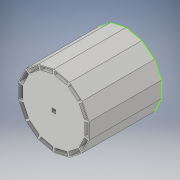
# Autodesk Inventor part: Magnetic Revolver
Saved by Autodesk Inventor 2018.3 (Build 223284000, 284)
## iProperties
Created: 2019-01-14
Part Number: Magnetic Revolver
Material: Generic
Document SubType Name: Modeling
Designer: locuser
Density: 1 g/cm^3
Appearance: Default
Author: locuser
Autodesk Inventor part; units mm, degrees
ref_plane "YZ Plane" through (0, 0, 0) normal (1, 0, 0) x (0, 1, 0)
ref_plane "XZ Plane" through (0, 0, 0) normal (0, 1, 0) x (-1, 0, 0)
ref_plane "XY Plane" through (0, 0, 0) normal (0, 0, 1) x (1, 0, 0)
sketch "Sketch1" plane through (0, 0, 0) normal (0, 0, 1) x (1, 0, 0)
  line L0 (0, 31.75) -> (13.7758, 28.6058)
  line L1 (13.7758, 28.6058) -> (24.8231, 19.7958)
  line L2 (24.8231, 19.7958) -> (30.954, 7.065)
  line L3 (30.954, 7.065) -> (30.954, -7.065)
  line L4 (30.954, -7.065) -> (24.8231, -19.7958)
  line L5 (24.8231, -19.7958) -> (13.7758, -28.6058)
  line L6 (13.7758, -28.6058) -> (0, -31.75)
  line L7 (0, -31.75) -> (-13.7758, -28.6058)
  line L8 (-13.7758, -28.6058) -> (-24.8231, -19.7958)
  line L9 (-24.8231, -19.7958) -> (-30.954, -7.065)
  line L10 (-30.954, -7.065) -> (-30.954, 7.065)
  line L11 (-30.954, 7.065) -> (-24.8231, 19.7958)
  line L12 (-24.8231, 19.7958) -> (-13.7758, 28.6058)
  line L13 (-13.7758, 28.6058) -> (0, 31.75)
  point P0 (0, 0)
  point P1 (0, 0)
  constraints: 28 end point, 1 coincident, 29 other
extrude "Extrusion1" add sketch "Sketch1" along normal blind 63.5
sketch "Sketch3" plane through (0, 0, 0) normal (0, 0, -1) x (-1, 0, 0)
  line L0 (0, -1.5875) -> (1.5875, -1.5875)
  line L1 (1.5875, -1.5875) -> (-1.5875, -1.5875)
  line L2 (1.5875, -1.5875) -> (-1.5875, -1.5875)
  line L3 (-1.5875, -1.5875) -> (-1.5875, 1.5921)
  line L4 (-1.5875, 1.5921) -> (1.5875, 1.5921)
  line L5 (1.5875, 1.5921) -> (1.5875, -1.5875)
  point P0 (0, 0)
  constraints: 12 end point, 2 horizontal, 2 parallel, 1 perpendicular, 1 point on line
extrude "Extrusion3" cut sketch "Sketch3" against normal blind 63.5
sketch "Sketch4" plane through (0, 0, 0) normal (0, 0, -1) x (-1, 0, 0)
  line L0 (-13.7758, 28.6058) -> (0, 31.75) projected
  line L1 (0, 0) -> (0, 31.75)
  line L2 (0, 31.75) -> (0, 0)
  line L3 (0, 26.7538) -> (11.6081, 24.1044)
  line L4 (11.6081, 24.1044) -> (20.917, 16.6807)
  line L5 (20.917, 16.6807) -> (26.0831, 5.9533)
  line L6 (26.0831, 5.9533) -> (26.0831, -5.9533)
  line L7 (26.0831, -5.9533) -> (20.917, -16.6807)
  line L8 (20.917, -16.6807) -> (11.6081, -24.1044)
  line L9 (11.6081, -24.1044) -> (0, -26.7538)
  line L10 (0, -26.7538) -> (-11.6081, -24.1044)
  line L11 (-11.6081, -24.1044) -> (-20.917, -16.6807)
  line L12 (-20.917, -16.6807) -> (-26.0831, -5.9533)
  line L13 (-26.0831, -5.9533) -> (-26.0831, 5.9533)
  line L14 (-26.0831, 5.9533) -> (-20.917, 16.6807)
  line L15 (-20.917, 16.6807) -> (-11.6081, 24.1044)
  line L16 (-11.6081, 24.1044) -> (0, 26.7538)
  line L17 (-10.8414, 24.2794) -> (-13.0091, 28.7808)
  line L18 (-14.3715, 28.0758) -> (-12.2229, 23.6141)
  constraints: 36 end point, 4 point on line, 2 coincident, 1 collinear, 1 parallel, 1 vertical, 29 other
sketch "Sketch5" plane through (0, 0, 63.5) normal (0, 0, 1) x (1, 0, 0)
  line L0 (0.8565, 27.7445) -> (0.8565, 30.7925)
  line L1 (-0.9215, 30.7777) -> (-0.9215, 27.7297)
  line L2 (-12.5635, 26.0885) -> (-13.3645, 25.7027) construction
  line L3 (-11.2337, 25.376) -> (-12.5635, 28.1205)
  line L4 (-14.164, 27.346) -> (-12.8356, 24.6045)
  line L5 (-22.6387, 18.0538) -> (-23.193, 17.3587) construction
  line L6 (-21.1314, 17.9888) -> (-23.5145, 19.8892)
  line L7 (-24.623, 18.4991) -> (-22.24, 16.5987)
  line L8 (-28.23, 6.4433) -> (-28.4278, 5.5766) construction
  line L9 (-30.2111, 5.9601) -> (-27.2395, 5.2819)
  line L10 (-28.23, -6.4433) -> (-28.4278, -5.5766) construction
  line L11 (-26.8318, -7.0637) -> (-29.8154, -7.717)
  line L12 (-30.2111, -5.9836) -> (-27.2395, -5.333)
  line L13 (12.5635, 26.0885) -> (11.7625, 26.474) construction
  line L14 (12.8362, 24.6041) -> (14.1581, 27.3507)
  line L15 (12.5562, 28.1221) -> (11.2344, 25.3758)
  line L16 (22.6387, 18.0538) -> (22.0844, 18.7488) construction
  line L17 (22.24, 16.5987) -> (24.623, 18.4991)
  line L18 (23.5145, 19.8892) -> (21.1314, 17.9888)
  line L19 (28.23, 6.4433) -> (28.0322, 7.31) construction
  line L20 (27.2395, 5.2855) -> (30.2111, 5.9836)
  line L21 (29.8154, 7.717) -> (26.8524, 7.021)
  line L22 (27.2481, -6.2448) -> (27.4459, -5.3781) construction
  line L23 (22.6387, -18.0538) -> (23.193, -17.3587) construction
  line L24 (21.1314, -17.9888) -> (23.5145, -19.8892)
  line L25 (24.623, -18.4991) -> (22.24, -16.5987)
  line L26 (12.5635, -26.0885) -> (13.3645, -25.7027) construction
  line L27 (11.2433, -25.3738) -> (12.533, -28.1274)
  line L28 (14.1215, -27.3799) -> (12.8255, -24.6126)
  line L29 (0, -28.956) -> (-0.889, -28.956) construction
  line L30 (0.8793, -27.7393) -> (0.8793, -30.7873)
  line L31 (-0.8987, -30.7829) -> (-0.8987, -27.7349)
  line L32 (-12.5635, -26.0885) -> (-13.3645, -25.7027) construction
  line L33 (-12.8255, -24.6126) -> (-12.8255, -24.6126)
  line L34 (-11.2433, -25.3738) -> (-12.5601, -28.1212)
  line L35 (-14.148, -27.3602) -> (-14.1434, -27.3624)
  line L36 (-14.1434, -27.3624) -> (-12.8255, -24.6126)
  line L37 (-22.6387, -18.0538) -> (-23.193, -17.3587) construction
  line L38 (-21.1314, -17.9888) -> (-23.5145, -19.8892)
  line L39 (-24.623, -18.4991) -> (-22.24, -16.5987)
  line L40 (0, 30.988) -> (13.4452, 27.9192)
  line L41 (13.4452, 27.9192) -> (24.2274, 19.3207)
  line L42 (24.2274, 19.3207) -> (30.2111, 6.8955)
  line L43 (30.2111, 6.8955) -> (30.2111, -6.8955)
  line L44 (30.2111, -6.8955) -> (24.2274, -19.3207)
  line L45 (24.2274, -19.3207) -> (13.4452, -27.9192)
  line L46 (13.4452, -27.9192) -> (0, -30.988)
  line L47 (0, -30.988) -> (-13.4452, -27.9192)
  line L48 (-13.4452, -27.9192) -> (-24.2274, -19.3207)
  line L49 (-24.2274, -19.3207) -> (-30.2111, -6.8955)
  line L50 (-30.2111, -6.8955) -> (-30.2111, 6.8955)
  line L51 (-30.2111, 6.8955) -> (-24.2274, 19.3207)
  line L52 (-24.2274, 19.3207) -> (-13.4452, 27.9192)
  line L53 (-13.4452, 27.9192) -> (0, 30.988)
  line L54 (0, 27.94) -> (12.1227, 25.1731)
  line L55 (12.1227, 25.1731) -> (21.8444, 17.4203)
  line L56 (21.8444, 17.4203) -> (27.2395, 6.2172)
  line L57 (27.2395, 6.2172) -> (27.2395, -6.2172)
  line L58 (27.2395, -6.2172) -> (21.8444, -17.4203)
  line L59 (21.8444, -17.4203) -> (12.1227, -25.1731)
  line L60 (12.1227, -25.1731) -> (0, -27.94)
  line L61 (0, -27.94) -> (-12.1227, -25.1731)
  line L62 (-12.1227, -25.1731) -> (-21.8444, -17.4203)
  line L63 (-21.8444, -17.4203) -> (-27.2395, -6.2172)
  line L64 (-27.2395, -6.2172) -> (-27.2395, 6.2172)
  line L65 (-27.2395, 6.2172) -> (-21.8444, 17.4203)
  line L66 (-21.8444, 17.4203) -> (-12.1227, 25.1731)
  line L67 (-12.1227, 25.1731) -> (0, 27.94)
  line L68 (29.7904, -7.7728) -> (29.7989, -7.7368)
  line L69 (30.2111, -6.0474) -> (27.2395, -5.331)
  line L70 (27.2529, -6.2237) -> (27.0551, -7.0904) construction
  line L71 (26.8424, -7.0419) -> (29.8584, -7.6278)
  line L72 (-26.8692, 6.9862) -> (-29.8408, 7.6644)
  point P0 (0, 0)
  point P1 (0, 0)
  point P2 (0, 0)
  constraints: 146 end point, 60 point on line, 13 parallel, 2 vertical, 1 coincident, 1 horizontal, 1 perpendicular, 58 other
extrude "Extrusion4" cut sketch "Sketch5" against normal blind 60.96 contours L0 L40 L15 L54 | L67 L3 L53 L1 | L14 L41 L18 L55 | L66 L6 L52 L4 | L17 L42 L21 L56 | L65 L72 L51 L7 | L20 L43 L69 L57 | L64 L12 L50 L9 | L71 L44 L25 L58 | L63 L39 L49 L11 | L24 L45 L28 L59 | L62 L36 L35 L48 L38 | L27 L46 L30 L60 | L61 L31 L47 L34
body "Solid1"
